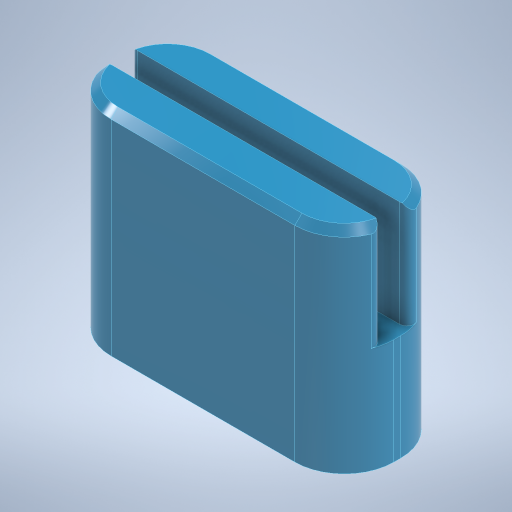
# Autodesk Inventor part: Base_MaterialRotativo
Saved by Autodesk Inventor 2024 (Build 280153000, 153)
## iProperties
Created: 2023-11-06
Part Number: Base_MaterialRotativo
Material: Generic
Document SubType Name: Modeling
Designer: fredy
Density: 1 g/cm^3
Appearance: Sky Blue Dark
Author: fredy
Autodesk Inventor part; units mm, degrees
ref_plane "YZ Plane" through (0, 0, 0) normal (1, 0, 0) x (0, 1, 0)
ref_plane "XZ Plane" through (0, 0, 0) normal (0, 1, 0) x (-1, 0, 0)
ref_plane "XY Plane" through (0, 0, 0) normal (0, 0, 1) x (1, 0, 0)
sketch "Sketch1" plane through (0, 0, 0) normal (0, 1, 0) x (-1, 0, 0)
  circle A0 centre (13.914, 0) radius 2.586
  line L0 (0, -5.46) -> (0, 5.46) projected
  circle A1 centre (-13.914, 0) radius 2.586
  circle A2 centre (0, 0) radius 3.9
  line L1 (14.1582, -2.5745) -> (0.3683, -3.8826)
  line L2 (-14.1582, -2.5745) -> (-0.3683, -3.8826)
  line L3 (23.1, 0) -> (-23.1, 0) projected
  line L4 (14.1582, 2.5745) -> (0.3683, 3.8826)
  line L5 (-14.1582, 2.5745) -> (-0.3683, 3.8826)
  circle A3 centre (14.5, 0) radius 0.75
  circle A4 centre (-14.5, 0) radius 0.75
  point P0 (14.1582, 2.5745)
  point P1 (0.3683, 3.8826)
  point P2 (-0.3683, 3.8826)
  point P3 (-14.1582, 2.5745)
  point P4 (-14.1582, -2.5745)
  point P5 (-0.3683, -3.8826)
  dimension "d0" = 5.1721
  dimension "d3" = 7.8
  dimension "d2" = 33
  dimension "d14" = 29
  dimension "d15" = 1.5
  constraints: 8 end point, 8 symmetric about line, 3 centre point, 2 horizontal alignment, 1 coincident, 10 other
  measures "d14" distance of A4.centre A3.centre
  measures "d15" diameter of A3
sketch "Sketch2" plane through (0, 0, 0) normal (0, 1, 0) x (-1, 0, 0)
  line L0 (-20, 7.5) -> (20, 7.5)
  line L1 (20, 7.5) -> (20, -7.5)
  line L2 (20, -7.5) -> (-20, -7.5)
  line L3 (-20, -7.5) -> (-20, 7.5)
  line L4 (-20, 7.5) -> (20, -7.5) construction
  line L5 (20, 7.5) -> (-20, -7.5) construction
  point P0 (0, 0)
  dimension "d4" = 40
  dimension "d5" = 15
  constraints: 12 end point, 2 midpoint, 2 parallel, 1 horizontal, 1 perpendicular
  measures "d4" distance of L0.start L0.end
  measures "d5" distance of L0.end L1.end
extrude "Extrusion1" add sketch "Sketch2" along normal blind 30
extrude "Extrusion2" cut sketch "Sketch1" along normal blind 4
fillet "Fillet1" radius 7 4 edges at (20, 15, 7.5) (20, 15, -7.5) (-20, 15, -7.5) (-20, 15, 7.5)
chamfer "Chamfer1" distance 1 angle 45 8 edges at (0, 30, -7.5) (-17.9497, 30, -5.4497) (-20, 30, 0) (-17.9497, 30, 5.4497) (0, 30, 7.5) (17.9497, 30, 5.4497) (20, 30, 0) (17.9497, 30, -5.4497)
extrude "Extrusion3" cut sketch "Sketch1" along normal blind 5 contours A3 L3 | L3 A3 | A4 L3 | L3 A4
sketch "Sketch4" plane through (0, 30, 0) normal (0, 1, 0) x (1, 0, 0)
  line L0 (-20, -1.8) -> (20, -1.8)
  line L1 (20, -1.8) -> (20, 1.8)
  line L2 (20, 1.8) -> (-20, 1.8)
  line L3 (-20, 1.8) -> (-20, -1.8)
  line L4 (-20, -1.8) -> (20, 1.8) construction
  line L5 (20, -1.8) -> (-20, 1.8) construction
  line L6 (15, 1.8) -> (5, 1.8)
  line L7 (5, 1.8) -> (5, -1.8)
  line L8 (5, -1.8) -> (15, -1.8)
  line L9 (15, -1.8) -> (15, 1.8)
  line L10 (15, 1.8) -> (5, -1.8) construction
  line L11 (5, 1.8) -> (15, -1.8) construction
  line L12 (0, 10.5) -> (0, -10.5) projected
  line L13 (-15, 1.8) -> (-5, 1.8)
  line L14 (-5, 1.8) -> (-5, -1.8)
  line L15 (-5, -1.8) -> (-15, -1.8)
  line L16 (-15, -1.8) -> (-15, 1.8)
  line L17 (-15, 1.8) -> (-5, -1.8) construction
  line L18 (-5, 1.8) -> (-15, -1.8) construction
  point P0 (0, 0)
  point P1 (0, 0)
  point P2 (10, 0)
  point P3 (-10, 0)
  point P4 (-10, 0)
  point P5 (-15, 1.8)
  point P6 (-15, -1.8)
  point P7 (-5, -1.8)
  point P8 (-5, 1.8)
  point P9 (15, -1.8)
  point P10 (15, 1.8)
  point P11 (5, 1.8)
  point P12 (5, -1.8)
  dimension "d23" = 3.6
  dimension "d24" = 40
  dimension "d33" = 3.6
  dimension "d34" = 10
  dimension "d35" = 20
  constraints: 36 end point, 5 midpoint, 5 symmetric about line, 4 parallel, 2 horizontal, 2 perpendicular, 1 coincident, 1 horizontal alignment
  measures "d23" distance of L2.end L0.start
  measures "d24" distance of L1.end L2.end
  measures "d33" distance of L6.end L7.end
  measures "d34" distance between parallel lines of L9 L7
  measures "d35" distance of point (-10, 0) point (10, 0)
extrude "Extrusion6" cut sketch "Sketch4" against normal blind 15
extrude "Extrusion7" cut sketch "Sketch4" against normal blind 25 contours L16 L2 L14 L0 | L7 L2 L9 L0
fillet "Fillet3" radius 1 4 edges at (19.8782, 22, 1.8) (19.8782, 22, -1.8) (-19.8782, 22, -1.8) (-19.8782, 22, 1.8)
body "Solid1"
